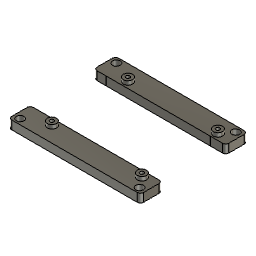
PiHddMateRails (Autodesk Fusion 360 design; units mm, degrees)
Autodesk Fusion 360 part; units mm, degrees
sketch "Sketch1" plane through (0, 0, 0) normal (0, 0, 1) x (1, 0, 0)
  line L0 (45, 34.5) -> (-40, 34.5)
  line L1 (-40, 34.5) -> (-40, -34.5)
  line L2 (-40, -34.5) -> (45, -34.5)
  line L3 (45, -34.5) -> (45, 34.5)
  circle A0 centre (41, 30.9952) radius 1.5
  line L4 (0, 56) -> (0, -61) construction
  line L5 (-71, -0.0048) -> (62, -0.0048) construction
  circle A1 centre (41, 30.9952) radius 2.5
  circle A2 centre (-36, 30.9952) radius 1.5
  circle A3 centre (-36, 30.9952) radius 2.5
  circle A4 centre (41, -31.0048) radius 1.5
  circle A5 centre (41, -31.0048) radius 2.5
  circle A6 centre (-36, -31.0048) radius 1.5
  circle A7 centre (-36, -31.0048) radius 2.5
  circle A8 centre (36, 24.4952) radius 1.25
  circle A9 centre (-22, 24.4952) radius 1.25
  circle A10 centre (36, -24.5048) radius 1.25
  circle A11 centre (-22, -24.5048) radius 1.25
  dimension "d1" = 85
  dimension "d2" = 69
  dimension "d3" = 3
  dimension "d8" = 5
  dimension "d13" = 2.5
  dimension "d14" = 24.5
  dimension "d17" = -58
  dimension "d18" = -49
  dimension "d45" = 41
  dimension "d46" = 41
  dimension "d47" = 41
  constraint horizontal L0
  constraint perpendicular L0 L1
  constraint parallel L0 L2
  constraint parallel L1 L3
  constraint perpendicular L0 L4
  constraint horizontal L5
  constraint concentric A0 A1
  measures "d1" distance of L1.end L2.end
  measures "d2" distance of L0.end L1.end
  measures "d3" diameter of A0
  measures "d8" diameter of A1
  measures "d13" diameter of A8
  measures "d14" distance of L5 A8.centre
  measures "d45" distance of A0.centre L4
  measures "d46" distance of L4 A4.centre
  measures "d47" distance of L4 A4.centre
extrude "Extrude1" add sketch "Sketch1" against normal blind 1.5 contours L0 L1 L2 L3 | A1 | A3 | A5 | A7 makes body 1
extrude "Extrude2" add sketch "Sketch1" along normal blind 4 contours L0 L1 L2 L3 bodies 1
fillet "Fillet1" radius 2 4 edges at (-40, -34.5, 1.25) (45, -34.5, 1.25) (45, 34.5, 1.25) (-40, 34.5, 1.25) on bodies 1
sketch "Sketch2" plane through (0, 0, 4) normal (0, 0, 1) x (-1, 0, 0)
  circle A0 centre (22, 24.5048) radius 1.25
  circle A1 centre (22, -24.4952) radius 1.25
  circle A2 centre (-36, 24.5048) radius 1.25
  circle A3 centre (-41, 31.0048) radius 2.5
  circle A4 centre (36, -30.9952) radius 2.5
  circle A5 centre (-36, -24.4952) radius 1.25
  circle A6 centre (36, 31.0048) radius 2.5
  circle A7 centre (-41, -30.9952) radius 2.5
  arc A8 (38, -34.5) -> (40, -32.5) centre (38, -32.5) ccw
  line L0 (40, -32.5) -> (40, 32.5)
  arc A9 (40, 32.5) -> (38, 34.5) centre (38, 32.5) ccw
  line L1 (38, 34.5) -> (-43, 34.5)
  arc A10 (-43, 34.5) -> (-45, 32.5) centre (-43, 32.5) ccw
  line L2 (-45, 32.5) -> (-45, -32.5)
  arc A11 (-45, -32.5) -> (-43, -34.5) centre (-43, -32.5) ccw
  line L3 (-43, -34.5) -> (38, -34.5)
  line L4 (34, -20.4952) -> (-37, -20.4952)
  line L5 (-37, -20.4952) -> (-37, 20.5048)
  line L6 (-37, 20.5048) -> (34, 20.5048)
  line L7 (34, 20.5048) -> (34, -20.4952)
  dimension "d28" = 4
  dimension "d29" = 6
  dimension "d30" = 8
  constraint horizontal L4
  constraint vertical L5
  constraint horizontal L6
  constraint vertical L7
  measures "d28" distance of A0.centre L6
  measures "d29" distance of L0 L7
  measures "d30" distance of L2 L5
extrude "Extrude3" cut sketch "Sketch2" against normal blind 5.5 contours L4 L5 L6 L7 bodies 1
fillet "Fillet2" radius 2 4 edges at (-34, 20.4952, 1.25) (-34, -20.5048, 1.25) (37, -20.5048, 1.25) (37, 20.4952, 1.25) on bodies 1
sketch "Sketch3" plane through (0, 0, 4) normal (0, 0, 1) x (-1, 0, 0)
  line L0 (-37, -18.4952) -> (-37, 18.5048)
  arc A0 (-35, 20.5048) -> (-37, 18.5048) centre (-35, 18.5048) ccw
  line L1 (-35, 20.5048) -> (32, 20.5048)
  arc A1 (34, 18.5048) -> (32, 20.5048) centre (32, 18.5048) ccw
  line L2 (34, 18.5048) -> (34, -18.4952)
  arc A2 (32, -20.4952) -> (34, -18.4952) centre (32, -18.4952) ccw
  line L3 (32, -20.4952) -> (-35, -20.4952)
  arc A3 (-37, -18.4952) -> (-35, -20.4952) centre (-35, -18.4952) ccw
  circle A4 centre (22, 24.5048) radius 1.25
  circle A5 centre (22, -24.4952) radius 1.25
  circle A6 centre (-36, 24.5048) radius 1.25
  circle A7 centre (-41, 31.0048) radius 2.5
  circle A8 centre (36, -30.9952) radius 2.5
  circle A9 centre (-36, -24.4952) radius 1.25
  circle A10 centre (36, 31.0048) radius 2.5
  circle A11 centre (-41, -30.9952) radius 2.5
  arc A12 (38, -34.5) -> (40, -32.5) centre (38, -32.5) ccw
  line L4 (40, -32.5) -> (40, 32.5)
  arc A13 (40, 32.5) -> (38, 34.5) centre (38, 32.5) ccw
  line L5 (38, 34.5) -> (-43, 34.5)
  arc A14 (-43, 34.5) -> (-45, 32.5) centre (-43, 32.5) ccw
  line L6 (-45, 32.5) -> (-45, -32.5)
  arc A15 (-45, -32.5) -> (-43, -34.5) centre (-43, -32.5) ccw
  line L7 (-43, -34.5) -> (38, -34.5)
  circle A16 centre (22, -24.4952) radius 3
  circle A17 centre (-36, -24.4952) radius 3
  circle A18 centre (22, 24.5048) radius 3
  circle A19 centre (-36, 24.5048) radius 3
  dimension "d35" = 6
  dimension "d38" = -58
  dimension "d39" = 49
  constraint concentric A5 A16
  measures "d35" diameter of A16
extrude "Extrude4" add sketch "Sketch3" along normal blind 2.5 contours A16 | A17 | A18 | A19 bodies 1
sketch "Sketch4" plane through (0, 0, 0) normal (0, 0, 1) x (1, 0, 0)
  line L0 (45, 20.4884) -> (-40, 20.4884)
  line L1 (-40, 20.4884) -> (-40, -20.4993)
  line L2 (-40, -20.4993) -> (45, -20.4993)
  line L3 (45, -20.4993) -> (45, 20.4884)
  line L4 (45, -32.5) -> (45, 32.5)
  line L5 (-40, 32.5) -> (-40, -32.5)
  constraint horizontal L0
  constraint perpendicular L0 L1
  constraint parallel L0 L2
  constraint parallel L1 L3
  constraint coincident L0.start L4
  constraint coincident L1.end L5
extrude "Extrude5" cut sketch "Sketch4" along normal up to surface (4 mm away) bodies 1
extrude "Extrude6" cut sketch "Sketch4" against normal up to surface (1.5 mm away) bodies 1 makes body 2 at (-6.5476, 30.7247, -1.5)
fillet "Fillet3" radius 2 3 edges at (45, -20.4993, 1.25) (-40, 20.4884, 1.25) (45, 20.4884, 1.25) on bodies 1 2
fillet "Fillet4" radius 2 1 edges at (-40, -20.4993, 1.25) on bodies 1
equation "d46 = d45"
equation "d47 = d45"
